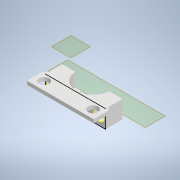
# Autodesk Inventor part: FrontPistonSupportTop
Saved by Autodesk Inventor 2022 (Build 260153000, 153)
## iProperties
Created: 2022-02-15
Part Number: FrontPistonSupportTop
Material: Generic
Document SubType Name: Modeling
Designer: siwat
Density: 1 g/cm^3
Appearance: Default
VLDS_Profile: Default Part
VLDS_TimeStamp: 2022-03-14
VLDS_FailCnt: 4
VLDS_AcceptCnt: 0
Author: siwat
Autodesk Inventor part; units mm, degrees
ref_plane "YZ Plane" through (0, 0, 0) normal (1, 0, 0) x (0, 1, 0)
ref_plane "XZ Plane" through (0, 0, 0) normal (0, 1, 0) x (-1, 0, 0)
ref_plane "Work Plane1" through (-68.3303, -5.5328, -24.5) normal (0, -1, 0) x (1, 0, 0)
sketch "Sketch1" plane through (-68.3303, -5.5328, -24.5) normal (0, -1, 0) x (1, 0, 0)
  line L0 (84, 20.5) -> (84, 5.3)
  line L1 (84, 5.3) -> (100, 5.3)
  line L2 (100, 5.3) -> (100, 0)
  line L3 (100, 0) -> (0, 0)
  line L4 (0, 0) -> (0, 5.3)
  line L5 (0, 5.3) -> (16, 5.3)
  line L6 (16, 5.3) -> (16, 20.5)
  line L7 (16, 20.5) -> (31.6697, 20.5)
  arc A0 (31.6697, 20.5) -> (68.3303, 20.5) centre (50, 25.5) ccw
  line L8 (68.3303, 20.5) -> (84, 20.5)
  circle A1 centre (50, 25.5) radius 19
  line L9 (69, 25.5) -> (84, 25.5)
  line L10 (84, 25.5) -> (84, 20.5)
  line L11 (31, 25.5) -> (16, 25.5)
  line L12 (16, 25.5) -> (16, 20.5)
  line L13 (84, 25.5) -> (84, 26.5)
  line L14 (84, 26.5) -> (68.9737, 26.5)
  line L15 (31.0263, 26.5) -> (16, 26.5)
  line L16 (16, 26.5) -> (16, 25.5)
  line L17 (84, 26.5) -> (84, 45.5)
  line L18 (84, 45.5) -> (16, 45.5)
  line L19 (16, 26.5) -> (16, 45.5)
  dimension "d0" = 1
  dimension "d1" = 20
  constraints: 40 end point, 6 horizontal, 6 perpendicular, 6 point on circle, 6 vertical, 4 point on line, 2 centre point, 2 line through centre, 1 coincident, 1 concentric, 11 other
  measures "d0" distance of L9.end L13.end
  measures "d1" distance from line of A1.centre L18
extrude "Extrusion1" add sketch "Sketch1" against normal blind 20 contours L14 A1 L15 L19 L18 L17
sketch "Sketch2" plane through (-52.3303, -5.5328, 21) normal (0, 0, 1) x (1, 0, 0)
  circle A0 centre (60.5, 10) radius 2.6
  circle A1 centre (7.5, 10) radius 2.6
  line L0 (0, 0) -> (0, 20) projected
  line L1 (68, 0) -> (68, 20) projected
  line L2 (68, 0) -> (0, 0) projected
  point P0 (52.3303, 5.5328)
  dimension "d4" = 5.2
  dimension "d5" = 5.2
  dimension "d6" = 7.5
  dimension "d7" = 7.5
  dimension "d8" = 10
  dimension "d9" = 10
  constraints: 2 centre point
  measures "d4" diameter of A0
  measures "d5" diameter of A1
  measures "d6" distance from line of L0 A1.centre
  measures "d7" distance from line of L1 A0.centre
  measures "d8" distance from line of L2 A0.centre
  measures "d9" distance from line of L2 A1.centre
extrude "Extrusion2" cut sketch "Sketch2" against normal through all
sketch "Sketch3" plane through (-68.3303, -5.5328, -24.5) normal (0, -1, 0) x (1, 0, 0)
  line L0 (16, 45.5) -> (84, 45.5) projected
  line L1 (16, 45.5) -> (84, 45.5)
  line L2 (84, 45.5) -> (84, 26.5)
  line L3 (84, 26.5) -> (16, 26.5)
  line L4 (16, 26.5) -> (16, 45.5)
  arc A0 (68.9737, 26.5) -> (31.0263, 26.5) centre (50, 25.5) ccw projected
  circle A1 centre (50, 25.5) radius 12.5
  point P0 (68.3303, 24.5)
  point P1 (84, 45.5)
  point P2 (37.5401, 26.5)
  point P3 (62.4599, 26.5)
  dimension "d14" = 25
  constraints: 8 end point, 2 parallel, 1 centre point, 1 coincident, 1 horizontal, 1 perpendicular
  measures "d14" diameter of A1
extrude "Extrusion3" add sketch "Sketch3" against normal blind 4.9 contours L0 L2 L3 A0 L4 | A0 L3 A1
sketch "Sketch4" plane through (-52.3303, -5.5328, 21) normal (0, 0, 1) x (1, 0, 0)
  circle A0 centre (60.5, 10) radius 2.6 projected
  circle A1 centre (60.5, 10) radius 5.75
  circle A2 centre (7.5, 10) radius 2.6 projected
  circle A3 centre (7.5, 10) radius 5.75
  point P0 (52.3303, 5.5328)
  dimension "d15" = 11.5
  dimension "d16" = 11.5
  constraints: 2 centre point, 2 coincident
  measures "d15" diameter of A1
  measures "d16" diameter of A3
extrude "Extrusion4" cut sketch "Sketch4" against normal blind 5
sketch "Sketch5" plane through (-52.3303, -5.5328, 21) normal (0, 0, 1) x (1, 0, 0)
  line L0 (46.4599, 0) -> (68, 0) projected
  line L1 (0, 20) -> (68, 20) projected
  line L2 (68, 0) -> (0, 0)
  line L3 (0, 0) -> (0, 20)
  line L4 (0, 20) -> (68, 20)
  line L5 (68, 20) -> (68, 0)
  circle A0 centre (60.5, 10) radius 5.75 projected
  circle A1 centre (7.5, 10) radius 5.75 projected
  point P0 (52.3303, 5.5328)
  constraints: 8 end point, 2 parallel, 1 horizontal, 1 perpendicular
sketch "Sketch7" plane through (-52.3303, 14.4672, 21) normal (0, 0, 1) x (1, 0, 0)
  line L0 (0, -20) -> (0, 0) projected
  line L1 (68, 0) -> (0, 0)
  line L2 (0, 0) -> (0, -4)
  line L3 (0, -4) -> (68, -4)
  line L4 (68, -4) -> (68, 0)
  point P0 (52.3303, -14.4672)
  dimension "d26" = 4
  constraints: 8 end point, 2 parallel, 1 horizontal, 1 perpendicular, 1 point on line
  measures "d26" distance between parallel lines of L1 L3
extrude "Extrusion6" add sketch "Sketch7" along normal blind 17
ref_plane "Work Plane2" through (-68.3303, 10.4672, -24) normal (0, -1, 0) x (1, 0, 0)
sketch "Sketch8" plane through (-68.3303, 10.4672, -24) normal (0, -1, 0) x (1, 0, 0)
  circle A0 centre (77.5, 52.7) radius 5.5
  circle A1 centre (22.5, 52.7) radius 5.5
  circle A2 centre (77.5, 52.7) radius 7.5
  circle A3 centre (22.5, 52.7) radius 7.5
  line L0 (77.5, 52.7) -> (22.5, 52.7)
  line L1 (16, 62.5) -> (84, 62.5) projected
  line L2 (84, 45.5) -> (84, 62.5) projected
  line L3 (16, 45.5) -> (16, 62.5) projected
  point P0 (68.3303, 24)
  dimension "d29" = 11
  dimension "d30" = 11
  dimension "d31" = 15
  dimension "d32" = 15
  dimension "d33" = 9.8
  dimension "d34" = 6.5
  dimension "d35" = 6.5
  constraints: 4 centre point, 2 coincident, 2 end point, 1 horizontal
  measures "d29" diameter of A0
  measures "d30" diameter of A1
  measures "d31" diameter of A2
  measures "d32" diameter of A3
  measures "d33" distance between parallel lines of L1 L0
  measures "d34" distance from line of A0.centre L2
  measures "d35" distance from line of L3 A1.centre
extrude "Extrusion7" cut sketch "Sketch8" against normal through all contours A0 | A1
sketch "Sketch9" plane through (-52.3303, 10.4672, 21) normal (0, -1, 0) x (1, 0, 0)
  line L0 (68, -19) -> (68, 17) projected
  line L1 (68, 17) -> (71.5, 17)
  line L2 (71.5, 17) -> (71.5, 0)
  line L3 (71.5, 0) -> (68, 0)
  line L4 (68, 0) -> (68, 17)
  line L5 (68, 0) -> (0, 0) projected
  line L6 (68, 17) -> (0, 17) projected
  line L7 (0, 17) -> (-3.5, 17)
  line L8 (-3.5, 17) -> (-3.5, 0)
  line L9 (-3.5, 0) -> (0, 0)
  line L10 (0, 0) -> (0, 17)
  point P0 (52.3303, -21)
  dimension "d44" = 3.5
  dimension "d45" = 3.5
  constraints: 16 end point, 4 parallel, 2 collinear, 2 horizontal, 2 perpendicular
  measures "d44" distance of L2.end L3.end
  measures "d45" distance of L9.end L8.end
ref_plane "Work Plane3" through (-54.8303, 14.449, -35) normal (0, -1, 0) x (1, 0, 0)
extrude "Extrusion8" add sketch "Sketch9" against normal up to surface (3.9818 mm away) contours L0 L1 L2 L3 | L9 L8 L7 L10
chamfer "Chamfer1" distance 3.5 angle 45 2 edges at (-52.3303, 12.4581, 21) (15.6697, 12.4581, 21)
equation "\"d15\" = d16"
body "Solid1"
